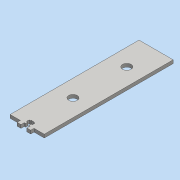
# Autodesk Inventor part: Y-Shaft-Holder-Front
Saved by Autodesk Inventor 2016 SP1 (Build 200210100, 210)
## iProperties
Created: 2016-01-21
Part Number: Y-Shaft-Holder-Front
Material: Generic
Document SubType Name: Modeling
Designer: Mohamed A.
Density: 1 g/cm^3
Appearance: Default
Author: Mohamed A.
Autodesk Inventor part; units mm, degrees
ref_plane "YZ Plane" through (0, 0, 0) normal (1, 0, 0) x (0, 1, 0)
ref_plane "XZ Plane" through (0, 0, 0) normal (0, 1, 0) x (-1, 0, 0)
ref_plane "XY Plane" through (0, 0, 0) normal (0, 0, 1) x (1, 0, 0)
sketch "Sketch1" plane through (0, 0, 0) normal (0, 0, 1) x (1, 0, 0)
  line L0 (-15.5, 60) -> (15.5, 60)
  line L1 (15.5, 60) -> (15.5, -57)
  line L2 (-15.5, -57) -> (-15.5, 60)
  line L3 (-15.5, 60) -> (15.5, -60) construction
  line L4 (15.5, 60) -> (-15.5, -60) construction
  line L5 (15.5, -57) -> (6.2, -57)
  line L6 (6.2, -57) -> (6.2, -60)
  line L7 (2.65, -60) -> (2.65, -57)
  line L8 (2.65, -57) -> (1.5, -57)
  line L9 (1.5, -57) -> (1.5, -55)
  line L10 (1.5, -55) -> (2.65, -55)
  line L11 (2.65, -55) -> (2.65, -52.6)
  line L12 (2.65, -52.6) -> (1.5, -52.6)
  line L13 (1.5, -52.6) -> (1.5, -52)
  line L14 (1.5, -52) -> (-1.5, -52)
  line L15 (-1.5, -52) -> (-1.5, -52.6)
  line L16 (-1.5, -52.6) -> (-2.65, -52.6)
  line L17 (-2.65, -52.6) -> (-2.65, -55)
  line L18 (-2.65, -55) -> (-1.5, -55)
  line L19 (-1.5, -57) -> (-2.65, -57)
  line L20 (-1.5, -55) -> (-1.5, -57)
  line L21 (-2.65, -57) -> (-2.65, -60)
  line L22 (-15.5, -57) -> (-6.2, -57)
  line L23 (-6.2, -57) -> (-6.2, -60)
  line L24 (0, -51.179) -> (0, -61.7681) construction
  line L25 (6.2, -60) -> (2.65, -60)
  line L26 (-2.65, -60) -> (-6.2, -60)
  line L27 (-24.2882, 0) -> (26.7754, 0) construction
  circle A0 centre (0, -15.4294) radius 3.9
  circle A1 centre (0, 33.4294) radius 3.9
  point P0 (0, 0)
  dimension "d0" = 31
  dimension "d4" = 3
  dimension "d6" = 3
  dimension "d7" = 2.4
  dimension "d10" = 5.3
  dimension "d11" = 8
  dimension "d12" = 5
  dimension "d13" = 12.4
  dimension "d14" = 7.8
  dimension "d15" = 44.5706
  dimension "d16" = 7.8
  dimension "d17" = 93.4294
  constraints: 56 end point, 13 perpendicular, 13 point on line, 7 horizontal, 5 vertical, 3 parallel, 2 centre point, 2 midpoint, 1 collinear, 6 other
  measures "d0" distance of L3.end L4.end
  measures "d4" distance of L6.end L5.end
  measures "d6" distance of L13.end L14.end
  measures "d7" distance of L10.end L11.end
  measures "d10" distance between parallel lines of L17 L11
  measures "d11" distance between parallel lines of L25 L14
  measures "d12" distance between parallel lines of L25 L10
  measures "d13" distance between parallel lines of L23 L6
  measures "d14" diameter of A0
  measures "d15" distance from line of L25 A0.centre
  measures "d16" diameter of A1
  measures "d17" distance from line of L25 A1.centre
extrude "Extrusion1" add sketch "Sketch1" along normal blind 3
equation "\"d13\" = 0.4 * d0"
body "Solid1"
